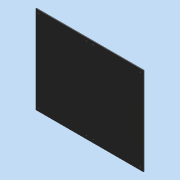
# Autodesk Inventor part: FrameBase
Saved by Autodesk Inventor 2016 (Build 200138000, 138)
## iProperties
Created: 2016-08-20
Part Number: FrameBase
Material: Dibond
Document SubType Name: Modeling
Designer: Sam
Density: 1 g/cm^3
Appearance: Generic
Author: Sam
Autodesk Inventor part; units mm, degrees
ref_plane "YZ Plane" through (0, 0, 0) normal (1, 0, 0) x (0, 1, 0)
ref_plane "XZ Plane" through (0, 0, 0) normal (0, 1, 0) x (-1, 0, 0)
ref_plane "XY Plane" through (0, 0, 0) normal (0, 0, 1) x (1, 0, 0)
sketch "Sketch1" plane through (0, 0, 0) normal (0, 1, 0) x (-1, 0, 0)
  line L0 (12, 9) -> (-428, 9)
  line L1 (-428, 9) -> (-428, -351)
  line L2 (-428, -351) -> (12, -351)
  line L3 (12, -351) -> (12, 9)
  point P0 (0, 0)
  dimension "d0" = 440
  dimension "d1" = 360
  constraints: 8 end point, 2 parallel, 1 horizontal, 1 perpendicular
  measures "d0" distance of L2.end L1.end
  measures "d1" distance of L1.end L0.end
extrude "Extrusion1" add sketch "Sketch1" along normal blind 3
hole "Hole1" at (0, 3, -3) direction (0, -1, 0) diameter 4 end through all
hole "Hole2" at (0, 3, -339) direction (0, -1, 0) diameter 4 end through all
hole "Hole3" at (416, 0, -3) direction (0, 1, 0) diameter 4 end through all
hole "Hole4" at (416, 0, -339) direction (0, 1, 0) diameter 4 end through all
hole "Hole5" at (194.5, 0, -339) direction (0, 1, 0) diameter 4 end through all
hole "Hole6" at (221.5, 0, -339) direction (0, 1, 0) diameter 4 end through all
hole "Hole7" at (194.5, 0, -3) direction (0, 1, 0) diameter 4 end through all
hole "Hole8" at (221.5, 0, -3) direction (0, 1, 0) diameter 4 end through all
body "Solid1"
